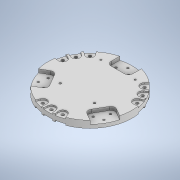
# Autodesk Inventor part: Body
Saved by Autodesk Inventor 2020.1 (Build 241239000, 239)
## iProperties
Created: 2022-03-03
Part Number: Body
Material: Generic
Document SubType Name: Modeling
Designer: OEM
Density: 1 g/cm^3
Appearance: Default
Author: OEM
Autodesk Inventor part; units mm, degrees
ref_plane "YZ Plane" through (0, 0, 0) normal (1, 0, 0) x (0, 1, 0)
ref_plane "XZ Plane" through (0, 0, 0) normal (0, 1, 0) x (-1, 0, 0)
ref_plane "XY Plane" through (0, 0, 0) normal (0, 0, 1) x (1, 0, 0)
sketch "Sketch1" plane through (0, 0, 0) normal (0, 1, 0) x (-1, 0, 0)
  circle A0 centre (0, 0) radius 60
  line L0 (133, 0) -> (-142, 0) construction
  line L1 (0, 144) -> (0, -175) construction
  line L2 (0, 0) -> (51.9615, 30) construction
  line L3 (0, 0) -> (-51.9615, 30) construction
  line L4 (15, -58.0948) -> (15, -43.0948) construction
  line L5 (15, -43.0948) -> (0, -43.0948) construction
  line L6 (-15, -58.0948) -> (-15, -43.0948) construction
  line L7 (-15, -43.0948) -> (0, -43.0948) construction
  line L8 (-15, -58.0948) -> (15, -43.0948) construction
  line L9 (-15, -43.0948) -> (15, -58.0948) construction
  circle A1 centre (9, -46.0948) radius 1.5
  circle A2 centre (-9, -46.0948) radius 1.5
  circle A3 centre (0, -54.0948) radius 1.5
  line L10 (15, -58.0948) -> (-15, -58.0948) construction
  circle A4 centre (-35.4192, 30.8416) radius 1.5
  circle A5 centre (-44.4192, 15.2531) radius 1.5
  circle A6 centre (-46.8474, 27.0474) radius 1.5
  circle A7 centre (44.4192, 15.2531) radius 1.5
  circle A8 centre (35.4192, 30.8416) radius 1.5
  circle A9 centre (46.8474, 27.0474) radius 1.5
  line L11 (-15.5, -57.9634) -> (-15.5, -39.5948)
  line L12 (-15.5, -39.5948) -> (0, -39.5948)
  line L13 (15.5, -57.9634) -> (15.5, -39.5948)
  line L14 (15.5, -39.5948) -> (0, -39.5948)
  line L15 (57.9477, 15.5583) -> (42.0401, 6.374)
  line L16 (42.0401, 6.374) -> (34.2901, 19.7974)
  line L17 (26.5401, 33.2208) -> (34.2901, 19.7974)
  line L18 (42.4477, 42.4051) -> (26.5401, 33.2208)
  line L19 (-42.4477, 42.4051) -> (-26.5401, 33.2208)
  line L20 (-26.5401, 33.2208) -> (-34.2901, 19.7974)
  line L21 (-42.0401, 6.374) -> (-34.2901, 19.7974)
  line L22 (-57.9477, 15.5583) -> (-42.0401, 6.374)
  circle A10 centre (24.5, -40) radius 1.25
  circle A11 centre (-24.5, -40) radius 1.25
  circle A12 centre (0, 55) radius 2
  circle A13 centre (0, 0) radius 55 construction
  circle A14 centre (14.235, 53.1259) radius 2
  circle A15 centre (24.5, 18) radius 1.5
  circle A16 centre (-24.5, 18) radius 1.5
  line L23 (21, 45) -> (-24.5, 45) construction
  circle A17 centre (-14.235, 53.1259) radius 2
  circle A18 centre (-53.1259, -14.235) radius 2
  circle A19 centre (-47.6314, -27.5) radius 2
  circle A20 centre (-38.8909, -38.8909) radius 2
  circle A21 centre (38.8909, -38.8909) radius 2
  circle A22 centre (47.6314, -27.5) radius 2
  circle A23 centre (53.1259, -14.235) radius 2
  arc A24 (6.2717, 59.6713) -> (-6.2717, 59.6713) centre (0, 0) ccw construction
  line L24 (0, 0) -> (60, 0) construction
  line L25 (5.7491, 54.6987) -> (6.2717, 59.6713)
  line L26 (5.7491, 54.6987) -> (0, 0) construction
  line L27 (-5.7491, 54.6987) -> (0, 0) construction
  line L28 (-5.7491, 54.6987) -> (-6.2717, 59.6713)
  arc A25 (-5.7491, 54.6987) -> (5.7491, 54.6987) centre (0, 55) ccw
  line L29 (-8.6039, 54.3229) -> (-9.3861, 59.2613)
  arc A26 (-19.7102, 51.3469) -> (-8.6039, 54.3229) centre (-14.235, 53.1259) ccw
  line L30 (-19.7102, 51.3469) -> (-21.5021, 56.0148)
  arc A27 (8.6039, 54.3229) -> (19.7102, 51.3469) centre (14.235, 53.1259) ccw
  line L31 (19.7102, 51.3469) -> (21.5021, 56.0148)
  line L32 (8.6039, 54.3229) -> (9.3861, 59.2613)
  arc A28 (-44.4959, -32.3282) -> (-50.245, -22.3705) centre (-47.6314, -27.5) ccw
  line L33 (-50.245, -22.3705) -> (-54.8127, -24.4042)
  line L34 (-44.4959, -32.3282) -> (-48.541, -35.2671)
  line L35 (-42.743, -34.6126) -> (-46.6288, -37.7592)
  arc A29 (-34.6126, -42.743) -> (-42.743, -34.6126) centre (-38.8909, -38.8909) ccw
  line L36 (-34.6126, -42.743) -> (-37.7592, -46.6288)
  line L37 (-51.3469, -19.7102) -> (-56.0148, -21.5021)
  arc A30 (-51.3469, -19.7102) -> (-54.3229, -8.6039) centre (-53.1259, -14.235) ccw
  line L38 (-54.3229, -8.6039) -> (-59.2613, -9.3861)
  arc A31 (50.245, -22.3705) -> (44.4959, -32.3282) centre (47.6314, -27.5) ccw
  line L39 (44.4959, -32.3282) -> (48.541, -35.2671)
  line L40 (50.245, -22.3705) -> (54.8127, -24.4042)
  line L41 (51.3469, -19.7102) -> (56.0148, -21.5021)
  arc A32 (54.3229, -8.6039) -> (51.3469, -19.7102) centre (53.1259, -14.235) ccw
  line L42 (54.3229, -8.6039) -> (59.2613, -9.3861)
  line L43 (42.743, -34.6126) -> (46.6288, -37.7592)
  arc A33 (42.743, -34.6126) -> (34.6126, -42.743) centre (38.8909, -38.8909) ccw
  line L44 (34.6126, -42.743) -> (37.7592, -46.6288)
  dimension "d0" = 120
  dimension "d2" = 120
  dimension "d3" = 15
  dimension "d6" = 3
  dimension "d7" = 3
  dimension "d9" = 3
  dimension "d10" = 11
  dimension "d14" = 15
  dimension "d15" = 6
  dimension "d18" = 360
  dimension "d24" = 6.5
  dimension "d25" = 6.5
  dimension "d28" = 360
  dimension "d39" = 2.5
  dimension "d40" = 24.5
  dimension "d41" = 40
  dimension "d44" = 4
  dimension "d46" = 110
  dimension "d47" = 4
  dimension "d48" = 15
  dimension "d51" = 58
  dimension "d52" = 85
  dimension "d55" = 360
  dimension "d59" = 6
  dimension "d62" = 15
  dimension "d66" = 345
  dimension "d70" = 360
  constraints: 90 end point, 33 centre point, 24 point on circle, 9 symmetric about line, 7 point on line, 4 coincident, 4 horizontal, 3 vertical, 2 perpendicular, 167 other
  measures "d2" angle of L2 L1
  measures "d3" distance between parallel lines of L4 L1
  measures "d6" diameter of A1
  measures "d7" distance from line of L5 A1.centre
  measures "d9" diameter of A3
  measures "d10" distance from line of L5 A3.centre
  measures "d14" distance of L4.start L4.end
  measures "d15" distance from line of L4 A1.centre
  measures "d24" distance from line of L11 A2.centre
  measures "d25" distance from line of L12 A2.centre
  measures "d39" diameter of A10
  measures "d40" distance from line of L1 A10.centre
  measures "d41" distance from line of L0 A10.centre
  measures "d44" diameter of A12
  measures "d46" diameter of A13
  measures "d47" diameter of A14
  measures "d51" distance of A15.centre A10.centre
  measures "d52" distance from line of L23 A10.centre
  measures "d59" angle of L26 L1
extrude "Extrusion1" add sketch "Sketch1" along normal blind 10 contours A0 L42 A32 L41 L40 A31 L39 L43 A33 L44 L13 L14 L12 L11 L36 A29 L35 L34 A28 L33 L37 A30 L38 L22 L21 L20 L19 L30 A26 L29 L28 A25 L25 L32 A27 L31 L18 L17 L16 L15
extrude "Extrusion3" add sketch "Sketch1" along normal blind 5 contours L15 L16 L17 L18 A0 | A0 L11 L12 L14 L13 | L19 L20 L21 L22 A0
extrude "Extrusion4" add sketch "Sketch1" along normal blind 8 contours A0 L41 A32 L42 | L31 A27 L32 A0 | A0 L39 A31 L40 | L25 A25 L28 A0 | A0 L44 A33 L43 | L29 A26 L30 A0 | A0 L35 A29 L36 | L38 A30 L37 A0 | A0 L33 A28 L34
extrude "Extrusion5" cut sketch "Sketch1" along normal blind 2 contours A0 L41 A32 L42 | L31 A27 L32 A0 | A0 L39 A31 L40 | L25 A25 L28 A0 | A0 L44 A33 L43 | L29 A26 L30 A0 | A0 L35 A29 L36 | L38 A30 L37 A0 | A0 L33 A28 L34
fillet "Fillet2" radius 6 6 edges at (-26.5401, 7.5, 33.2208) (-42.0401, 7.5, 6.374) (-15.5, 7.5, -39.5948) (15.5, 7.5, -39.5948) (42.0401, 7.5, 6.374) (26.5401, 7.5, 33.2208)
equation "\"d9\" = d6"
equation "\"d25\" = d24"
equation "\"d47\" = d44"
body "Solid1"
